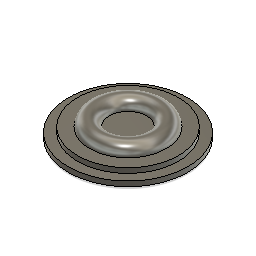
тортик_1 v1 (Autodesk Fusion 360 design; units mm, degrees)
Autodesk Fusion 360 part; units mm, degrees
note: some values were not read from the file. Chosen so that the rebuilt part matches the saved one: a setting.
cylinder "CylinderPrimitive1" add diameter 122.066 height 5 placed x (1, 0, 0) y (0, 0, -1) z (0, 1, 0) at (0, 0, 0)
sketch "Sketch2" plane through (0, 0, 0) normal (0, 1, 0) x (1, 0, 0)
torus "TorusPrimitive1" add centre line diameter 100 section diameter 5 placed x (1, 0, 0) y (0, 0, -1) z (0, 1, 0) at (0, 0, 0)
cylinder "CylinderPrimitive2" add diameter 102.956 height 5 placed x (1, 0, 0) y (0, 0, -1) z (0, 1, 0) at (0, 5, 0)
torus "TorusPrimitive2" add centre line diameter 58.102 section diameter 20 placed x (-1, 0, 0) y (0, 0, 1) z (0, 1, 0) at (0, 10, 0)
